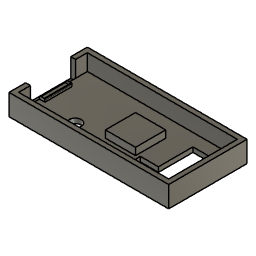
top (Autodesk Fusion 360 design; units mm, degrees)
Autodesk Fusion 360 part; units mm, degrees
sketch "Skizze1" plane through (0, 0, 0) normal (0, 0, 1) x (1, 0, 0)
  line L0 (0, 0) -> (53, 0)
  line L1 (53, 0) -> (53, 26)
  line L2 (53, 26) -> (0, 26)
  line L3 (0, 26) -> (0, 0)
  line L4 (1.6, 1.6) -> (51.4, 1.6)
  line L5 (51.4, 1.6) -> (51.4, 24.4)
  line L6 (51.4, 24.4) -> (1.6, 24.4)
  line L7 (1.6, 24.4) -> (1.6, 1.6)
  line L8 (3.4, 3.4) -> (49.6, 3.4)
  line L9 (49.6, 3.4) -> (49.6, 22.6)
  line L10 (49.6, 22.6) -> (3.4, 22.6)
  line L11 (3.4, 22.6) -> (3.4, 3.4)
  circle A0 centre (14.4, 7.6) radius 2
  line L12 (40.8, 20.25) -> (49.6, 20.25)
  line L13 (49.6, 20.25) -> (49.6, 5.75)
  line L14 (49.6, 5.75) -> (40.8, 5.75)
  line L15 (40.8, 5.75) -> (40.8, 20.25)
  line L16 (34.3, 22.6) -> (40.4, 22.6)
  line L17 (3.4, 8.5) -> (1.6, 8.5)
  line L18 (1.6, 8.5) -> (1.6, 17.5)
  line L19 (1.6, 17.5) -> (3.4, 17.5)
  line L20 (3.4, 17.5) -> (3.4, 8.5)
  line L21 (23.8, 8.2) -> (33.8, 8.2)
  line L22 (33.8, 8.2) -> (33.8, 18.2)
  line L23 (33.8, 18.2) -> (23.8, 18.2)
  line L24 (23.8, 18.2) -> (23.8, 8.2)
  line L25 (34.8, 1.6) -> (42.3, 1.6)
  line L26 (42.3, 1.6) -> (42.3, 8.8)
  line L27 (42.3, 8.8) -> (34.8, 8.8)
  line L28 (34.8, 8.8) -> (34.8, 1.6)
  dimension "d1" = 46.2
  dimension "d2" = 19.2
  dimension "d3" = 1.6
  dimension "d4" = 1.8
  dimension "d5" = 1.6
  dimension "d6" = 1.8
  dimension "d7" = 1.8
  dimension "d8" = 1.6
  dimension "d9" = 1.8
  dimension "d10" = 1.6
  dimension "d20" = 4
  dimension "d21" = 12.8
  dimension "d26" = 14.5
  dimension "d29" = 6
  dimension "d34" = 8.8
  dimension "d35" = 9
  dimension "d45" = 10
  dimension "d46" = 10
  dimension "d47" = 15.8
  dimension "d48" = 4.8
  dimension "d51" = 9.1
  dimension "d52" = 7.5
  dimension "d53" = 7.2
  constraint horizontal L0
  constraint vertical L1
  constraint horizontal L2
  constraint vertical L3
  constraint coincident L0.start L3.end
  constraint horizontal L4
  constraint vertical L5
  constraint horizontal L6
  constraint vertical L7
  constraint horizontal L8
  constraint vertical L9
  constraint horizontal L10
  constraint vertical L11
  constraint horizontal L12
  constraint vertical L13
  constraint horizontal L14
  constraint vertical L15
  constraint horizontal L16
  constraint coincident L10 L16.start
  constraint coincident L9 L12.end
  constraint midpoint L9 L13
  constraint horizontal L17
  constraint vertical L18
  constraint horizontal L19
  constraint vertical L20
  constraint coincident L7 L18.end
  constraint coincident L11 L17.start
  constraint midpoint L11 L20
  constraint horizontal L21
  constraint vertical L22
  constraint horizontal L23
  constraint vertical L24
  constraint horizontal L25
  constraint vertical L26
  constraint horizontal L27
  constraint vertical L28
  constraint coincident L4 L25.start
  measures "d1" distance of L9 L11
  measures "d2" distance of L8 L10
  measures "d3" distance of L0 L4
  measures "d4" distance of L4 L8
  measures "d5" distance of L3 L7
  measures "d6" distance of L7 L11
  measures "d7" distance of L6 L10
  measures "d8" distance of L2 L6
  measures "d9" distance of L5 L9
  measures "d10" distance of L1 L5
  measures "d20" diameter of A0
  measures "d21" distance of L7 A0.centre
  measures "d26" distance of L12 L14
  measures "d29" distance of L4 A0.centre
  measures "d34" distance of L13 L15
  measures "d35" distance of L17 L19
  measures "d45" distance of L21.start L21.end
  measures "d46" distance of L21 L23
  measures "d47" distance of L9 L22
  measures "d48" distance of L8 L21
  measures "d51" distance of L5 L26
  measures "d52" distance of L26 L28
  measures "d53" distance of L4 L27
extrude "Extrusion1" add sketch "Skizze1" along normal blind 1.6 contours L0 L1 L2 L3 | L4 L7 L8 L11 L17 L28 | L4 L8 L25 L26 L28 | L7 L11 L17 L18 L19 L20 | L4 L5 L6 L7 L8 L9 L10 L11 L13 L16 L19 L26 | L8 L14 L15 L26 L27 L28 | L8 L9 L10 L11 L12 L15 L16 L20 L27 L28 | L8 L9 L14 L26 | L9 L12 L13 L14 L15 L26 L27 | L14 L15 L26 L27 | A0 | L21 L22 L23 L24
extrude "Extrusion2" add sketch "Skizze1" along normal blind 7 contours L0 L1 L2 L3
ref_plane "Arbeitsebene1" through (0, 13, 3.5) normal (-1, 0, 0) x (0, -1, 0)
sketch "Skizze2" plane through (0, 0, 0) normal (-1, 0, 0) x (0, -1, 0)
  line L0 (-20.5, 7) -> (-5.5, 7)
  line L1 (-5.5, 7) -> (-5.5, 0.8)
  line L2 (-5.5, 0.8) -> (-20.5, 0.8)
  line L3 (-20.5, 0.8) -> (-20.5, 7)
  line L4 (-26, 7) -> (0, 7)
  line L5 (-26, 0) -> (0, 0)
  dimension "d16" = 0.8
  dimension "d17" = 15
  constraint horizontal L0
  constraint vertical L1
  constraint horizontal L2
  constraint vertical L3
  constraint coincident L0.start L4
  constraint midpoint L0 L4
  measures "d16" distance of L2 L5
  measures "d17" distance of L1 L3
extrude "Extrusion3" cut sketch "Skizze2" against normal blind 1.6
extrude "Extrusion4" cut sketch "Skizze1" along normal blind 1.6 contours L4 L8 L25 L26 L28 | L8 L14 L15 L26 L27 L28 | L9 L12 L13 L14 L15 L26 L27 | L14 L15 L26 L27 | A0
extrude "Extrusion5" add sketch "Skizze1" along normal blind 2.6 contours L7 L11 L17 L18 L19 L20
ref_plane "Arbeitsebene2" through (1.6, 13, 1.7) normal (-1, 0, 0) x (0, 0, 1)
sketch "Skizze3" plane through (1.6, 0, 0) normal (-1, 0, 0) x (0, -1, 0)
  line L0 (-8.5, 2.6) -> (-17.5, 2.6)
  line L1 (-17, 2.1) -> (-9, 2.1)
  line L2 (-17.5, 2.6) -> (-8.5, 2.6)
  arc A0 (-9, 2.1) -> (-8.5, 2.6) centre (-9, 2.6) ccw
  arc A1 (-17.5, 2.6) -> (-17, 2.1) centre (-17, 2.6) ccw
  dimension "d39" = 0.5
  dimension "d41" = 0.5
  dimension "d42" = 0.5
  constraint horizontal L0
  constraint horizontal L1
  constraint coincident L0.start L2
  constraint tangent L1 A0
  constraint coincident L0.start L2.end
  constraint tangent L1 A1
  constraint coincident L0.end L2.start
  measures "d39" distance of L0 L1
  measures "d41" radius of A0
  measures "d42" radius of A1
extrude "Extrusion6" cut sketch "Skizze3" against normal blind 1.6
extrude "Extrusion7" add sketch "Skizze1" along normal blind 4 contours L21 L22 L23 L24
equation "d13 = 5.4 mm + 1.6 mm"
equation "d36 = 1.6 mm + 0.5 mm + 0.5 mm"
equation "d53 = 1.7 mm + 5.5 mm"
